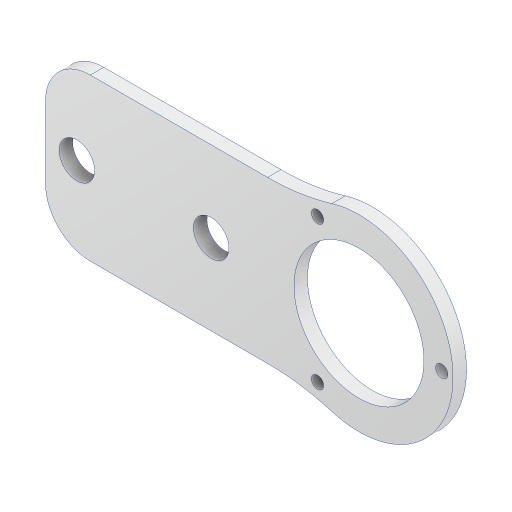
# Autodesk Inventor part: wrist_pitch_plate
Saved by Autodesk Inventor 2024.3 (Build 283343000, 343)
## iProperties
Created: 2024-10-12
Part Number: wrist_pitch_plate
Material: アルミニウム 6061
Document SubType Name: Sheet Metal
Designer: haya
Density: 2.7 g/cm^3
Sheet Metal Rule: Default_mm
Appearance: アルミニウム - フラット
Mass: 24.1844 g
Surface Area: 70.3203 cm^2
Volume: 8.95719 cm^3
Author: haya
Autodesk Inventor part; units mm, degrees
ref_plane "YZ Plane" through (0, 0, 0) normal (1, 0, 0) x (0, 1, 0)
ref_plane "XZ Plane" through (0, 0, 0) normal (0, 1, 0) x (-1, 0, 0)
ref_plane "XY Plane" through (0, 0, 0) normal (0, 0, 1) x (1, 0, 0)
sketch "スケッチ1" plane through (0, 0, 0) normal (0, 0, 1) x (1, 0, 0)
  line L0 (-30, 18) -> (30, 18)
  line L1 (30, 18) -> (30, -18)
  line L2 (30, -18) -> (-30, -18)
  line L3 (-30, -18) -> (-30, 18)
  line L4 (0, 0) -> (0, 18) construction
  line L5 (0, 0) -> (30, 0) construction
  dimension "d0" = 36
  dimension "d1" = 60
  measures "d0" distance of L0.end L1.end
  measures "d1" distance of L0.start L0.end
extrude "プレート1" add sketch "スケッチ1" along normal blind 3
sketch "スケッチ13" plane through (0, 0, 0) normal (0, 0, -1) x (-1, 0, 0)
  line L0 (0, 0) -> (30, 0) construction
  line L1 (30, -18) -> (30, 18) projected
  line L2 (-30, 18) -> (-30, -18) projected
  point P0 (23, 0)
  point P1 (-7, 0)
  dimension "d127" = 30
  dimension "d129" = 7
  constraints: 2 end point, 2 point on line, 1 midpoint
  measures "d127" distance of point (23, 0) point (-7, 0)
  measures "d129" distance from line of point (23, 0) L1
hole "穴10" at (-23, 0, 0) at (7, 0, 0) direction (0, 0, 1) diameter 7.9 depth 3
sketch "スケッチ15" plane through (0, 0, 0) normal (0, 0, -1) x (-1, 0, 0)
  circle A0 centre (-40, 0) radius 21
  line L0 (-30, -18) -> (-30, 18) projected
  point P0 (0, 0)
  dimension "d130" = 42
  dimension "d131" = 10
  constraints: 1 centre point
  measures "d130" diameter of A0
  measures "d131" distance from line of A0.centre L0
extrude "押し出し1" add sketch "スケッチ15" against normal up to surface (3 mm away)
fillet "フィレット1" radius 10 2 edges at (-30, 18, 1.5) (-30, -18, 1.5)
sketch "スケッチ16" plane through (0, 0, 0) normal (0, 0, -1) x (-1, 0, 0)
  arc A0 (-29.1833, 18) -> (-29.1833, -18) centre (-40, 0) ccw projected
  circle A1 centre (-40, 0) radius 14.5
  point P0 (0, 0)
  dimension "d134" = 29
  constraints: 1 centre point, 1 coincident
  measures "d134" diameter of A1
extrude "押し出し2" cut sketch "スケッチ16" against normal up to surface (3 mm away)
sketch "スケッチ17" plane through (0, 0, 0) normal (0, 0, -1) x (-1, 0, 0)
  circle A0 centre (-40, 0) radius 14.5 projected
  line L0 (-40, 0) -> (-61, 0) construction
  arc A1 (-29.1833, 18) -> (-29.1833, -18) centre (-40, 0) ccw projected
  point P0 (0, 0)
  point P1 (-58.5, 0)
  point P2 (-30.75, -16.0215)
  point P3 (-30.75, 16.0215)
  dimension "d137" = 18.5
  dimension "d140" = 360
  constraints: 2 end point, 1 horizontal, 1 point on circle, 1 point on line, 4 other
  measures "d137" distance of point (-58.5, 0) L0.start
hole "穴11" at (58.5, 0, 0) at (30.75, -16.0215, 0) at (30.75, 16.0215, 0) direction (0, 0, 1) diameter 2.7 depth 3
fillet "フィレット3" radius 50 2 edges at (29.1833, 18, 1.5) (29.1833, -18, 1.5)
equation "\"d125\" = Thickness"
equation "\"d147\" = Thickness"
equation "\"d2\" = Thickness"
equation "\"BendRadius\" = Thickness"
equation "\"BendReliefWidth\" = Thickness"
equation "\"BendReliefDepth\" = 0.5 * Thickness"
equation "\"CornerReliefSize\" = 4 * Thickness"
equation "\"MinimumRemnant\" = 2 * Thickness"
equation "\"TransitionRadius\" = BendRadius"
equation "\"JacobiRadiusSize\" = BendRadius"
equation "\"GapSize\" = Thickness"
equation "\"Thickness\" = 3"
